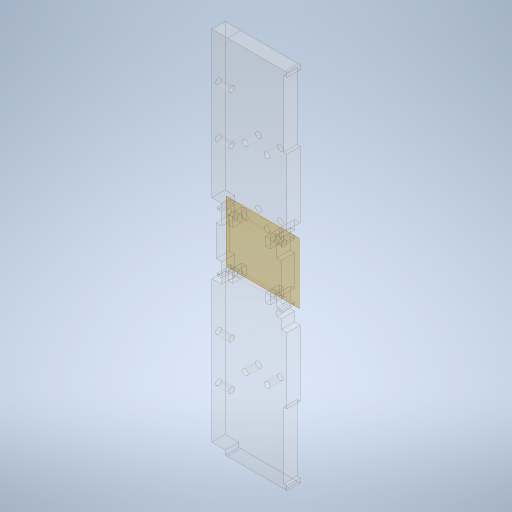
# Autodesk Inventor part: _face_froward_2
Saved by Autodesk Inventor 2024.3 (Build 283343000, 343)
## iProperties
Created: 2024-09-09
Part Number: _face_froward_2
Material: PMMA 플라스틱
Document SubType Name: Modeling
Designer: gretc
Density: 1.188 g/cm^3
Appearance: 폴리카보네이트 - 선명
Author: gretc
Autodesk Inventor part; units mm, degrees
ref_plane "YZ Plane" through (0, 0, 0) normal (1, 0, 0) x (0, 1, 0)
ref_plane "XZ Plane" through (0, 0, 0) normal (0, 1, 0) x (-1, 0, 0)
ref_plane "작업 평면1" through (31.9, -59, 0) normal (0, 0, 1) x (0, 1, 0)
ref_plane "작업 평면2" through (31.9, -59, 0) normal (0, 0, 1) x (0, 1, 0)
sketch "스케치2" plane through (31.9, -59, 0) normal (0, 0, 1) x (0, 1, 0)
  line L0 (27, 33) -> (27, 8) projected
  line L1 (25.6003, 33) -> (27, 33) projected
  line L2 (25.3997, 33) -> (25.6003, 33) projected
  line L3 (21.525, 33) -> (25.3997, 33) projected
  line L4 (21.525, 35.5) -> (21.525, 33) projected
  line L5 (7.475, 35.5) -> (21.525, 35.5) projected
  line L6 (7.475, 35.5) -> (7.475, 33) projected
  line L7 (3.6003, 33) -> (7.475, 33) projected
  line L8 (3.3997, 33) -> (3.6003, 33) projected
  line L9 (2, 33) -> (3.3997, 33) projected
  line L10 (2, 33) -> (2, 8) projected
  line L11 (2, 8) -> (3.3997, 8) projected
  line L12 (3.3997, 8) -> (3.6003, 8) projected
  line L13 (3.6003, 8) -> (7.475, 8) projected
  line L14 (7.475, 5.5) -> (7.475, 8) projected
  line L15 (7.475, 5.5) -> (21.525, 5.5) projected
  line L16 (21.525, 5.5) -> (21.525, 8) projected
  line L17 (21.525, 8) -> (25.3997, 8) projected
  line L18 (25.3997, 8) -> (25.6003, 8) projected
  line L19 (25.6003, 8) -> (27, 8) projected
  line L20 (96.5, 31.3414) -> (94.5, 31.3414) projected
  line L21 (94.5, 31.3414) -> (94.5, 29.9) projected
  line L22 (94.5, 29.9) -> (64.5, 29.9) projected
  line L23 (64.5, 29.9) -> (64.5, 31.3414) projected
  line L24 (64.5, 31.3414) -> (62.5, 31.3414) projected
  line L25 (62.5, 31.3414) -> (62.5, 25.05) projected
  line L26 (62.5, 9.75) -> (62.5, 25.05) projected
  line L27 (62.5, 9.75) -> (62.5, 3.4586) projected
  line L28 (64.5, 3.4586) -> (62.5, 3.4586) projected
  line L29 (64.5, 3.4586) -> (64.5, 4.9) projected
  line L30 (94.5, 4.9) -> (64.5, 4.9) projected
  line L31 (94.5, 4.9) -> (94.5, 3.4586) projected
  line L32 (96.5, 3.4586) -> (94.5, 3.4586) projected
  line L33 (96.5, 3.4586) -> (96.5, 4.4) projected
  line L34 (96.5, 4.4) -> (98, 4.4) projected
  line L35 (98, 30.4) -> (98, 4.4) projected
  line L36 (98, 30.4) -> (96.5, 30.4) projected
  line L37 (96.5, 30.4) -> (96.5, 31.3414) projected
  line L38 (-67.5, 3.4586) -> (-65.5, 3.4586) projected
  line L39 (-65.5, 3.4586) -> (-65.5, 4.9) projected
  line L40 (-65.5, 4.9) -> (-35.5, 4.9) projected
  line L41 (-35.5, 4.9) -> (-35.5, 3.4586) projected
  line L42 (-35.5, 3.4586) -> (-33.5, 3.4586) projected
  line L43 (-33.5, 3.4586) -> (-33.5, 9.75) projected
  line L44 (-33.5, 25.05) -> (-33.5, 9.75) projected
  line L45 (-33.5, 25.05) -> (-33.5, 31.3414) projected
  line L46 (-35.5, 31.3414) -> (-33.5, 31.3414) projected
  line L47 (-35.5, 31.3414) -> (-35.5, 29.9) projected
  line L48 (-65.5, 29.9) -> (-35.5, 29.9) projected
  line L49 (-65.5, 29.9) -> (-65.5, 31.3414) projected
  line L50 (-67.5, 31.3414) -> (-65.5, 31.3414) projected
  line L51 (-67.5, 31.3414) -> (-67.5, 30.4) projected
  line L52 (-67.5, 30.4) -> (-69, 30.4) projected
  line L53 (-69, 4.4) -> (-69, 30.4) projected
  line L54 (-69, 4.4) -> (-67.5, 4.4) projected
  line L55 (-67.5, 4.4) -> (-67.5, 3.4586) projected
  line L56 (27.9121, 35) -> (27.9121, 37.5) projected
  line L57 (1.0879, 37.5) -> (27.9121, 37.5) projected
  line L58 (1.0879, 37.5) -> (1.0879, 35) projected
  line L59 (1.0879, 35) -> (5.975, 35) projected
  line L60 (5.975, 33) -> (5.975, 35) projected
  line L61 (5.975, 33) -> (7.475, 33) projected
  line L62 (7.475, 33) -> (7.475, 35.5) projected
  line L63 (7.475, 35.5) -> (21.525, 35.5) projected
  line L64 (21.525, 33) -> (21.525, 35.5) projected
  line L65 (21.525, 33) -> (23.025, 33) projected
  line L66 (23.025, 33) -> (23.025, 35) projected
  line L67 (23.025, 35) -> (27.9121, 35) projected
  line L68 (27.9121, 3.5) -> (27.9121, 6) projected
  line L69 (23.025, 6) -> (27.9121, 6) projected
  line L70 (23.025, 8) -> (23.025, 6) projected
  line L71 (21.525, 8) -> (23.025, 8) projected
  line L72 (21.525, 8) -> (21.525, 5.5) projected
  line L73 (7.475, 5.5) -> (21.525, 5.5) projected
  line L74 (7.475, 8) -> (7.475, 5.5) projected
  line L75 (5.975, 8) -> (7.475, 8) projected
  line L76 (5.975, 8) -> (5.975, 6) projected
  line L77 (1.0879, 6) -> (5.975, 6) projected
  line L78 (1.0879, 6) -> (1.0879, 3.5) projected
  line L79 (1.0879, 3.5) -> (27.9121, 3.5) projected
  line L80 (27, 33) -> (27, 35)
  line L81 (2, 33) -> (2, 35)
  line L82 (2, 8) -> (2, 6)
  line L83 (27, 8) -> (27, 6)
  line L84 (-33.5, 3.4586) -> (-33.5, 31.3414)
  line L85 (-33.5, 31.3414) -> (1.0879, 31.3414)
  line L86 (1.0879, 31.3414) -> (1.0879, 3.4586)
  line L87 (1.0879, 3.4586) -> (-33.5, 3.4586)
  line L88 (1.0879, 31.3414) -> (2, 31.3414)
  line L89 (2, 31.3414) -> (2, 6)
  line L90 (2, 6) -> (1.0879, 6)
  line L91 (1.0879, 6) -> (1.0879, 31.3414)
  line L92 (62.5, 3.4586) -> (62.5, 31.3414)
  line L93 (62.5, 31.3414) -> (27.9121, 31.3414)
  line L94 (27.9121, 31.3414) -> (27.9121, 3.4586)
  line L95 (27.9121, 3.4586) -> (62.5, 3.4586)
  line L96 (27.9121, 35) -> (27.9121, 31.3414)
  line L97 (27.9121, 31.3414) -> (27.9121, 35)
  line L98 (27.9121, 35) -> (62.5, 35)
  line L99 (62.5, 35) -> (62.5, 31.3414)
  line L100 (62.5, 31.3414) -> (27.9121, 31.3414)
  line L101 (2, 31.3414) -> (2, 35)
  line L102 (2, 35) -> (-33.5, 35)
  line L103 (-33.5, 35) -> (-33.5, 31.3414)
  line L104 (-33.5, 31.3414) -> (2, 31.3414)
  point P0 (59, 31.9)
  point P1 (1.0879, 3.5)
  point P2 (27.9121, 3.5)
  point P3 (1.0879, 35)
  constraints: 50 end point, 11 parallel, 8 point on line, 7 perpendicular, 2 collinear, 2 vertical
extrude "돌출1" add sketch "스케치2" along normal blind 6 contours L80 L67 L96 L94 L69 L83 L0 | L0 L19 L18 L17 L16 L15 L14 L13 L12 L11 L10 L9 L8 L7 L6 L5 L4 L3 L2 L1 | L98 L99 L93 L96 | L94 L93 L25 L26 L27 L95 L68 | L24 L23 L22 L21 L20 L37 L36 L35 L34 L33 L32 L31 L30 L29 L28 L27 L26 L25 | L86 L87 L43 L44 L45 L85 L78 | L59 L81 L10 L88 L85 L103 L102 | L86 L88 L10 L82 L77 | L42 L41 L40 L39 L38 L55 L54 L53 L52 L51 L50 L49 L48 L47 L46 L45 L44 L43
sketch "스케치4" plane through (31.9, -59, 6) normal (0, 0, 1) x (1, 0, 0)
  line L0 (-6, 34.6) -> (-3.5, 34.6) projected
  line L1 (-6, -5.6) -> (-3.5, -5.6) projected
  line L2 (-37.5, -5.6) -> (-35, -5.6) projected
  line L3 (-3.5, 34.6) -> (-6, 34.6)
  line L4 (-6, 34.6) -> (-6, 27.9121)
  line L5 (-6, 27.9121) -> (-3.5, 27.9121)
  line L6 (-3.5, 27.9121) -> (-3.5, 34.6)
  line L7 (-3.5, -5.6) -> (-6, -5.6)
  line L8 (-6, -5.6) -> (-6, 1.0804)
  line L9 (-6, 1.0804) -> (-3.5, 1.0804)
  line L10 (-3.5, 1.0804) -> (-3.5, -5.6)
  line L11 (-3.4586, -35.5) -> (-3.4586, 1.0879) projected
  line L12 (-6, -5.6) -> (-3.4586, -5.6)
  line L13 (-3.4586, -5.6) -> (-3.4586, 34.6)
  line L14 (-3.4586, 34.6) -> (-6, 34.6)
  line L15 (-6, 34.6) -> (-6, -5.6)
  point P0 (-31.9, 59)
  point P1 (-6, 27.9121)
  point P2 (-6, 1.0804)
  point P3 (-3.5, -5.6)
  point P4 (-3.4586, 1.0879)
  point P5 (-3.5, 34.6)
  constraints: 24 end point, 6 parallel, 4 perpendicular, 2 point on line, 1 horizontal
extrude "돌출2" cut sketch "스케치4" against normal blind 6
sketch "스케치5" plane through (31.9, -59, 6) normal (0, 0, 1) x (1, 0, 0)
  line L0 (-8, 28.9421) -> (-6, 28.9421) projected
  line L1 (-6, 30.3929) -> (-3.5, 30.3929) projected
  line L2 (-6, -1.3929) -> (-3.5, -1.3929) projected
  line L3 (-6, 1.0879) -> (-3.5, 1.0879) projected
  line L4 (-35, 27.9121) -> (-37.5, 27.9121) projected
  line L5 (-37.5, 30.3929) -> (-35, 30.3929) projected
  line L6 (-37.5, 1.0879) -> (-35, 1.0879) projected
  line L7 (-37.5, -1.3929) -> (-35, -1.3929) projected
  line L8 (-3.5, 27.9121) -> (-6, 27.9121) projected
  line L9 (-35, 30.3929) -> (-35, 27.9121)
  line L10 (-35, 27.9121) -> (-33, 27.9121)
  line L11 (-33, 27.9121) -> (-33, 30.3929)
  line L12 (-33, 30.3929) -> (-35, 30.3929)
  line L13 (-35, 62.5) -> (-35, 27) projected
  line L14 (-6, 27.9121) -> (-6, 30.3929)
  line L15 (-6, 30.3929) -> (-8, 30.3929)
  line L16 (-8, 30.3929) -> (-8, 27.9121)
  line L17 (-8, 27.9121) -> (-6, 27.9121)
  line L18 (-6, 1.0879) -> (-6, -1.3929)
  line L19 (-6, -1.3929) -> (-8, -1.3929)
  line L20 (-8, -1.3929) -> (-8, 1.0879)
  line L21 (-8, 1.0879) -> (-6, 1.0879)
  line L22 (-35, -1.3929) -> (-35, 1.0879)
  line L23 (-35, 1.0879) -> (-33, 1.0879)
  line L24 (-33, 1.0879) -> (-33, -1.3929)
  line L25 (-33, -1.3929) -> (-35, -1.3929)
  point P0 (-31.9, 59)
  dimension "d4" = 2
  dimension "d5" = 2
  constraints: 32 end point, 8 parallel, 7 perpendicular, 1 collinear
  measures "d4" distance of L10.end L4.start
  measures "d5" distance of L15.end L1.start
extrude "돌출3" cut sketch "스케치5" against normal blind 6
sketch "스케치6" plane through (23.9, -37.475, 0) normal (1, 0, 0) x (0, 0, -1)
  circle A0 centre (-2.8, 3.975) radius 1.35 projected
  circle A1 centre (-2.8, -18.025) radius 1.35 projected
  point P0 (0, 37.475)
extrude "돌출4" cut sketch "스케치6" against normal up to surface (25 mm away)
sketch "스케치7" plane through (31.9, -59, 6) normal (0, 0, 1) x (1, 0, 0)
  line L0 (-8, 26.85) -> (-33, 26.85) projected
  line L1 (-8, 24.15) -> (-33, 24.15) projected
  line L2 (-8, 4.85) -> (-33, 4.85) projected
  line L3 (-8, 2.15) -> (-33, 2.15) projected
  line L4 (-33, 26.85) -> (-33, 24.15)
  line L5 (-33, 24.15) -> (-29, 24.15)
  line L6 (-29, 24.15) -> (-29, 26.85)
  line L7 (-29, 26.85) -> (-33, 26.85)
  line L8 (-33, 27) -> (-33, 21.525) projected
  line L9 (-33, 2.15) -> (-33, 4.85)
  line L10 (-33, 4.85) -> (-29, 4.85)
  line L11 (-29, 4.85) -> (-29, 2.15)
  line L12 (-29, 2.15) -> (-33, 2.15)
  line L13 (-8, 4.85) -> (-8, 2.15)
  line L14 (-8, 2.15) -> (-12, 2.15)
  line L15 (-12, 2.15) -> (-12, 4.85)
  line L16 (-12, 4.85) -> (-8, 4.85)
  line L17 (-8, 26.85) -> (-8, 24.15)
  line L18 (-8, 24.15) -> (-12, 24.15)
  line L19 (-12, 24.15) -> (-12, 26.85)
  line L20 (-12, 26.85) -> (-8, 26.85)
  line L21 (-13, 27.5) -> (-13, 23.5)
  line L22 (-13, 23.5) -> (-11, 23.5)
  line L23 (-11, 23.5) -> (-11, 27.5)
  line L24 (-11, 27.5) -> (-13, 27.5)
  line L25 (-13, 27.5) -> (-11, 23.5) construction
  line L26 (-13, 23.5) -> (-11, 27.5) construction
  line L27 (-30, 27.5) -> (-30, 23.5)
  line L28 (-30, 23.5) -> (-28, 23.5)
  line L29 (-28, 23.5) -> (-28, 27.5)
  line L30 (-28, 27.5) -> (-30, 27.5)
  line L31 (-30, 27.5) -> (-28, 23.5) construction
  line L32 (-30, 23.5) -> (-28, 27.5) construction
  line L33 (-11, 1.5) -> (-11, 5.5)
  line L34 (-11, 5.5) -> (-13, 5.5)
  line L35 (-13, 5.5) -> (-13, 1.5)
  line L36 (-13, 1.5) -> (-11, 1.5)
  line L37 (-11, 1.5) -> (-13, 5.5) construction
  line L38 (-11, 5.5) -> (-13, 1.5) construction
  line L39 (-30, 1.5) -> (-30, 5.5)
  line L40 (-30, 5.5) -> (-28, 5.5)
  line L41 (-28, 5.5) -> (-28, 1.5)
  line L42 (-28, 1.5) -> (-30, 1.5)
  line L43 (-30, 1.5) -> (-28, 5.5) construction
  line L44 (-30, 5.5) -> (-28, 1.5) construction
  point P0 (-31.9, 59)
  point P1 (-12, 25.5)
  point P2 (-29, 25.5)
  point P3 (-12, 3.5)
  point P4 (-29, 3.5)
  dimension "d10" = 4
  dimension "d11" = 4
  dimension "d12" = 4
  dimension "d13" = 4
  dimension "d14" = 4
  dimension "d15" = 2
  dimension "d16" = 4
  dimension "d17" = 2
  dimension "d18" = 4
  constraints: 80 end point, 16 parallel, 12 midpoint, 12 perpendicular, 1 collinear
  measures "d10" distance of L5.end L1.end
  measures "d11" distance of L2.end L10.end
  measures "d12" distance of L3.start L14.end
  measures "d13" distance of L1.start L18.end
  measures "d14" distance of L21.start L21.end
  measures "d15" distance of L22.end L21.end
  measures "d16" distance of L27.start L27.end
  measures "d17" distance of L28.end L27.end
  measures "d18" distance of L33.start L33.end
extrude "돌출5" cut sketch "스케치7" against normal blind 10 contours L23 L1 L19 L0 | L0 L21 L24 L23 | L19 L1 L21 L0 | L23 L22 L21 L1 | L29 L1 L6 L0 | L0 L27 L30 L29 | L6 L1 L27 L0 | L29 L28 L27 L1 | L33 L3 L15 L2 | L2 L35 L34 L33 | L15 L3 L35 L2 | L33 L36 L35 L3 | L41 L3 L11 L2 | L2 L39 L40 L41 | L11 L3 L39 L2 | L41 L42 L39 L3
sketch "스케치8" plane through (1.5, -128, 0) normal (0, -1, 0) x (1, 0, 0)
  line L0 (0, 0) -> (26, 0) projected
  line L1 (26, 0) -> (26, 6) projected
  line L2 (0, 6) -> (26, 6) projected
  line L3 (0, 0) -> (0, 6) projected
  line L4 (-0.9414, 0) -> (0, 0) projected
  line L5 (0, 0) -> (0, 6) projected
  line L6 (-0.9414, 6) -> (0, 6) projected
  line L7 (-0.9414, 0) -> (-0.9414, 6) projected
  line L8 (26, 0) -> (26.9414, 0) projected
  line L9 (26.9414, 0) -> (26.9414, 6) projected
  line L10 (26, 6) -> (26.9414, 6) projected
  line L11 (26, 0) -> (26, 6) projected
  point P0 (-1.5, 0)
  point P1 (26, 0)
extrude "돌출6" cut sketch "스케치8" against normal blind 1.5
sketch "스케치9" plane through (1.5, 39, 0) normal (0, 1, 0) x (1, 0, 0)
  line L0 (26, 0) -> (0, 0) projected
  line L1 (0, 0) -> (0, -6) projected
  line L2 (26, -6) -> (0, -6) projected
  line L3 (26, 0) -> (26, -6) projected
  line L4 (26.9414, 0) -> (26, 0) projected
  line L5 (26, 0) -> (26, -6) projected
  line L6 (26.9414, -6) -> (26, -6) projected
  line L7 (26.9414, 0) -> (26.9414, -6) projected
  line L8 (0, 0) -> (0, -6) projected
  line L9 (0, 0) -> (-0.9414, 0) projected
  line L10 (-0.9414, 0) -> (-0.9414, -6) projected
  line L11 (0, -6) -> (-0.9414, -6) projected
  line L12 (0, 0) -> (0, -6) projected
  point P0 (-1.5, 0)
  point P1 (26, 0)
extrude "돌출7" cut sketch "스케치9" against normal blind 1.5
ref_plane "작업 평면3" through (-5.6, -126.5, -61.0993) normal (1, 0, 0) x (0, 1, 0)
sketch "스케치10" plane through (2, -124.5, 0) normal (-1, 0, 0) x (0, 0, 1)
  line L0 (0, 30) -> (0, 0)
  line L1 (0, 0) -> (6, 0)
  line L2 (6, 30) -> (6, 0)
  line L3 (0, 30) -> (6, 30)
  line L4 (0, 32) -> (0, 30)
  line L5 (0, 30) -> (6, 30)
  line L6 (6, 32) -> (6, 30)
  line L7 (0, 32) -> (6, 32)
  line L8 (6, 64.1071) -> (0, 64.1071)
  line L9 (0, 64.1071) -> (0, 32)
  line L10 (0, 32) -> (6, 32)
  line L11 (6, 64.1071) -> (6, 32)
  line L12 (0, 160) -> (0, 130)
  line L13 (0, 130) -> (6, 130)
  line L14 (6, 160) -> (6, 130)
  line L15 (0, 160) -> (6, 160)
  line L16 (0, 162) -> (0, 160)
  line L17 (0, 160) -> (6, 160)
  line L18 (6, 162) -> (6, 160)
  line L19 (0, 162) -> (6, 162)
  line L20 (0, 130) -> (0, 128)
  line L21 (0, 128) -> (6, 128)
  line L22 (6, 130) -> (6, 128)
  line L23 (0, 130) -> (6, 130)
  line L24 (0, 95.8929) -> (6, 95.8929)
  line L25 (6, 128) -> (6, 95.8929)
  line L26 (0, 128) -> (6, 128)
  line L27 (0, 128) -> (0, 95.8929)
  point P0 (0, 124.5)
  point P1 (0, 160)
  point P2 (0, 128)
  point P3 (0, 30)
extrude "돌출8" add sketch "스케치10" along normal up to surface (7.6 mm away)
sketch "스케치11" plane through (-5.6, -124.5, 0) normal (-1, 0, 0) x (0, 0, 1)
  circle A0 centre (3, 22) radius 1.35 projected
  circle A1 centre (3, 117.8929) radius 1.35 projected
  circle A2 centre (3, 42.1071) radius 1.35 projected
  circle A3 centre (3, 140) radius 1.35 projected
  line L0 (12.0993, -2) -> (12.0993, 162) projected
  line L1 (12.0993, 162) -> (-61.0993, 162) projected
  line L2 (-61.0993, 162) -> (-61.0993, -2) projected
  line L3 (-61.0993, -2) -> (12.0993, -2) projected
  line L4 (0, 88.15) -> (0, 71.85) projected
  arc A4 (-1, 70.85) -> (0, 71.85) centre (-1, 71.85) ccw projected
  line L5 (-1, 70.85) -> (-3, 70.85) projected
  arc A5 (-3, 70.85) -> (-5.35, 68.5) centre (-3, 68.5) ccw projected
  line L6 (-5.35, 68.5) -> (-5.35, 66.5) projected
  arc A6 (-6.35, 65.5) -> (-5.35, 66.5) centre (-6.35, 66.5) ccw projected
  line L7 (-6.35, 65.5) -> (-49.15, 65.5) projected
  arc A7 (-50.15, 66.5) -> (-49.15, 65.5) centre (-49.15, 66.5) ccw projected
  line L8 (-50.15, 66.5) -> (-50.15, 68.5) projected
  arc A8 (-50.15, 68.5) -> (-52.5, 70.85) centre (-52.5, 68.5) ccw projected
  line L9 (-52.5, 70.85) -> (-54, 70.85) projected
  arc A9 (-55.5, 72.35) -> (-54, 70.85) centre (-54, 72.35) ccw projected
  line L10 (-55.5, 72.35) -> (-55.5, 87.65) projected
  arc A10 (-54, 89.15) -> (-55.5, 87.65) centre (-54, 87.65) ccw projected
  line L11 (-54, 89.15) -> (-52.5, 89.15) projected
  arc A11 (-52.5, 89.15) -> (-50.15, 91.5) centre (-52.5, 91.5) ccw projected
  line L12 (-50.15, 91.5) -> (-50.15, 93.5) projected
  arc A12 (-49.15, 94.5) -> (-50.15, 93.5) centre (-49.15, 93.5) ccw projected
  line L13 (-49.15, 94.5) -> (-6.35, 94.5) projected
  arc A13 (-5.35, 93.5) -> (-6.35, 94.5) centre (-6.35, 93.5) ccw projected
  line L14 (-5.35, 93.5) -> (-5.35, 91.5) projected
  arc A14 (-5.35, 91.5) -> (-3, 89.15) centre (-3, 91.5) ccw projected
  line L15 (-3, 89.15) -> (-1, 89.15) projected
  arc A15 (0, 88.15) -> (-1, 89.15) centre (-1, 88.15) ccw projected
  circle A16 centre (-24.5, 97.3) radius 1.35 projected
  circle A17 centre (-2.5, 97.3) radius 1.35 projected
  circle A18 centre (2.8, 91) radius 1.35 projected
  circle A19 centre (-46.5, 97.3) radius 1.35 projected
  circle A20 centre (-24.5, 62.7) radius 1.35 projected
  circle A21 centre (2.8, 69) radius 1.35 projected
  circle A22 centre (-46.5, 62.7) radius 1.35 projected
  circle A23 centre (-2.5, 62.7) radius 1.35 projected
  point P0 (0, 124.5)
extrude "돌출9" cut sketch "스케치11" against normal blind 6 contours A0 | A1 | A2 | A3
sketch "스케치12" plane through (31.9, -59, 6) normal (0, 0, 1) x (1, 0, 0)
  line L0 (-31.3414, -27.5) -> (-3.4586, -27.5) projected
  line L1 (-31.3414, -33.5) -> (-3.4586, -33.5) projected
  line L2 (-3.4586, -33.5) -> (-31.3414, -33.5)
  line L3 (-31.3414, -33.5) -> (-31.3414, 0.0092)
  line L4 (-31.3414, 0.0092) -> (-3.4586, 0.0092)
  line L5 (-3.4586, 0.0092) -> (-3.4586, -33.5)
  line L6 (-31.3414, 0.0092) -> (-3.4586, 0.0092)
  line L7 (-3.4586, 0.0092) -> (-3.4586, 33.5184)
  line L8 (-3.4586, 33.5184) -> (-31.3414, 33.5184)
  line L9 (-31.3414, 33.5184) -> (-31.3414, 0.0092)
  line L10 (-3.4586, 33.5184) -> (-31.3414, 33.5184)
  line L11 (-31.3414, 33.5184) -> (-31.3414, 27.5184)
  line L12 (-31.3414, 27.5184) -> (-3.4586, 27.5184)
  line L13 (-3.4586, 27.5184) -> (-3.4586, 33.5184)
  line L14 (-31.3414, -33.5) -> (-22.3414, -33.5)
  line L15 (-3.4586, -33.5) -> (-12.4586, -33.5)
  line L16 (-12.4586, -33.5) -> (-22.3414, -33.5)
  line L17 (-22.3414, -33.5) -> (-22.3414, -30.5)
  line L18 (-22.3414, -30.5) -> (-12.4586, -30.5)
  line L19 (-12.4586, -30.5) -> (-12.4586, -33.5)
  line L20 (-3.4586, 30.5184) -> (-31.3414, 30.5184)
  line L21 (-12.4586, -30.5) -> (-22.3414, -30.5)
  line L22 (-22.3414, -30.5) -> (-22.3414, 30.5184)
  line L23 (-22.3414, 30.5184) -> (-12.4586, 30.5184)
  line L24 (-12.4586, 30.5184) -> (-12.4586, -30.5)
  circle A0 centre (-22.3414, -30.5) radius 1.35
  circle A1 centre (-12.4586, -30.5) radius 1.35
  circle A2 centre (-22.3414, 30.5184) radius 1.35
  circle A3 centre (-12.4586, 30.5184) radius 1.35
  point P0 (-31.9, 59)
  dimension "d29" = 33.5092
  dimension "d30" = 33.5092
  dimension "d31" = 6
  dimension "d32" = 9
  dimension "d33" = 9
  dimension "d34" = 3
  dimension "d35" = 2.7
  dimension "d36" = 2.7
  dimension "d37" = 2.7
  dimension "d38" = 2.7
  constraints: 46 end point, 10 parallel, 5 perpendicular, 4 centre point, 4 coincident, 3 collinear, 2 horizontal, 2 midpoint, 2 point on line
  measures "d29" distance of L3.end L1.start
  measures "d30" distance of L7.end L4.end
  measures "d31" distance of L11.end L8.end
  measures "d32" distance of L1.start L14.end
  measures "d33" distance of L1.end L15.end
  measures "d34" distance of L14.end L17.end
  measures "d35" diameter of A0
  measures "d36" diameter of A1
  measures "d37" diameter of A2
  measures "d38" diameter of A3
extrude "돌출10" cut sketch "스케치12" against normal blind 6 contours A0 L18 L22 | L22 L17 A0 | A1 L19 L24 | L24 L18 A1 | L18 A0 L17 | L19 A1 L18 | A2 L20 L22 | L22 L20 A2 | A2 L20 | A3 L20 L24 | L24 L20 A3 | L20 A3
sketch "스케치13" plane through (31.9, -59, 6) normal (0, 0, 1) x (1, 0, 0)
  line L0 (-9.7174, 59) -> (-25.0826, 59)
  circle A0 centre (-12.4586, 59.5) radius 1.35 projected
  circle A1 centre (-22.3414, 59.5) radius 1.35 projected
  point P0 (-31.9, 59)
  constraints: 2 end point, 1 horizontal, 2 other
extrude "돌출11" cut sketch "스케치13" against normal blind 6
